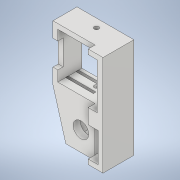
# Autodesk Inventor part: 30_Mount_Nema_Motor_attachement_for_XYstage_v3
Saved by Autodesk Inventor 2022.3 (Build 263350000, 350)
## iProperties
Created: 2021-05-10
Part Number: 30_Mount_Nema_Motor_attachement_for_XYstage_v3
Material: Generic
Document SubType Name: Modeling
Designer: diederichbenedict
Density: 1 g/cm^3
Appearance: Smooth - White
Author: diederichbenedict
Autodesk Inventor part; units mm, degrees
ref_plane "YZ Plane" through (0, 0, 0) normal (1, 0, 0) x (0, 1, 0)
sketch "Sketch1" plane through (0, 0, 0) normal (0, 0, 1) x (1, 0, 0)
  arc A0 (-7.9, -11.4) -> (-11.4, -7.9) centre (-11.4, -11.4) ccw projected
  line L0 (-7.9, -11.4) -> (-7.9, -13.5) projected
  line L1 (7.9, -13.5) -> (-7.9, -13.5) projected
  line L2 (7.9, -13.5) -> (7.9, -11.4) projected
  arc A1 (11.4, -7.9) -> (7.9, -11.4) centre (11.4, -11.4) ccw projected
  line L3 (11.4, -7.9) -> (13.5, -7.9) projected
  line L4 (13.5, 7.9) -> (13.5, -7.9) projected
  line L5 (13.5, 7.9) -> (11.4, 7.9) projected
  arc A2 (7.9, 11.4) -> (11.4, 7.9) centre (11.4, 11.4) ccw projected
  line L6 (7.9, 11.4) -> (7.9, 13.5) projected
  line L7 (-7.9, 13.5) -> (7.9, 13.5) projected
  line L8 (-7.9, 13.5) -> (-7.9, 11.4) projected
  arc A3 (-11.4, 7.9) -> (-7.9, 11.4) centre (-11.4, 11.4) ccw projected
  line L9 (-11.4, 7.9) -> (-13.5, 7.9) projected
  line L10 (-13.5, -7.9) -> (-13.5, 7.9) projected
  line L11 (-13.5, -7.9) -> (-11.4, -7.9) projected
  circle A4 centre (0, 0) radius 2.5 projected
  circle A5 centre (11.5, -26.7) radius 1.75 projected
  circle A6 centre (11.5, -38.3) radius 1.75 projected
  line L12 (14.7, -41.5) -> (14.7, -23.5) projected
  line L13 (14.7, -23.5) -> (8.7, -23.5) projected
  line L14 (8.7, -23.5) -> (8.7, -41.5) projected
  line L15 (8.7, -41.5) -> (14.7, -41.5) projected
  line L16 (-14, -11.5) -> (-14, -8.9) projected
  arc A7 (-14, -11.5) -> (-11.5, -14) centre (-11.5, -11.5) ccw projected
  line L17 (-8.9, -14) -> (-11.5, -14) projected
  line L18 (-8.9, -14) -> (-8.9, -11.4) projected
  arc A8 (-8.9, -11.4) -> (-11.4, -8.9) centre (-11.4, -11.4) ccw projected
  line L19 (-11.4, -8.9) -> (-14, -8.9) projected
  circle A9 centre (-11.5, -11.5) radius 1.1 projected
  arc A10 (-11.4, 8.9) -> (-8.9, 11.4) centre (-11.4, 11.4) ccw projected
  line L20 (-8.9, 11.4) -> (-8.9, 14) projected
  line L21 (-11.5, 14) -> (-8.9, 14) projected
  arc A11 (-11.5, 14) -> (-14, 11.5) centre (-11.5, 11.5) ccw projected
  line L22 (-14, 8.9) -> (-14, 11.5) projected
  line L23 (-14, 8.9) -> (-11.4, 8.9) projected
  circle A12 centre (-11.5, 11.5) radius 1.1 projected
  arc A13 (14, 11.5) -> (11.5, 14) centre (11.5, 11.5) ccw projected
  line L24 (14, 11.5) -> (14, 8.9) projected
  arc A14 (14, 11.5) -> (11.5, 14) centre (11.5, 11.5) ccw projected
  line L25 (8.9, 14) -> (11.5, 14) projected
  line L26 (8.9, 14) -> (8.9, 11.4) projected
  arc A15 (8.9, 11.4) -> (11.4, 8.9) centre (11.4, 11.4) ccw projected
  line L27 (11.4, 8.9) -> (14, 8.9) projected
  circle A16 centre (11.5, 11.5) radius 1.1 projected
  arc A17 (11.4, -8.9) -> (8.9, -11.4) centre (11.4, -11.4) ccw projected
  line L28 (8.9, -11.4) -> (8.9, -14) projected
  line L29 (11.5, -14) -> (8.9, -14) projected
  arc A18 (11.5, -14) -> (14, -11.5) centre (11.5, -11.5) ccw projected
  line L30 (14, -8.9) -> (14, -11.5) projected
  line L31 (14, -8.9) -> (11.4, -8.9) projected
  circle A19 centre (11.5, -11.5) radius 1.1 projected
  line L32 (8.6, -41.6) -> (8.6, -23.4)
  line L33 (8.6, -23.4) -> (14.8, -23.4)
  line L34 (14.8, -23.4) -> (14.8, -41.6)
  line L35 (14.8, -41.6) -> (8.6, -41.6)
  line L36 (-14, -14) -> (14, -14)
  line L37 (14, -14) -> (14, 13.7431)
  line L38 (14, 13.7431) -> (-14, 13.7431)
  line L39 (-14, 13.7431) -> (-14, -14)
  line L40 (-14.2, -14.2) -> (14.2, -14.2)
  line L41 (14.2, -14.2) -> (14.2, 13.9431)
  line L42 (14.2, 13.9431) -> (-14.2, 13.9431)
  line L43 (-14.2, 13.9431) -> (-14.2, -14.2)
  line L44 (-17.2, 17) -> (17.8, 17)
  line L45 (17.8, 17) -> (17.8, -44.6)
  line L46 (17.8, -44.6) -> (-9.3, -44.6)
  line L47 (-17.2, -17.2) -> (-17.2, 17)
  line L48 (-17.2, -17.2) -> (-9.3, -44.6)
  circle A20 centre (0, -32.5) radius 4.8 construction
  line L49 (8.7, -23.5) -> (-6.3, -23.5) construction
  line L50 (-6.3, -41.5) -> (-6.3, -23.5) construction
  line L51 (-6.3, -41.5) -> (8.7, -41.5) construction
  line L52 (8.7, -23.5) -> (8.7, -41.5) construction
  circle A21 centre (0, -32.5) radius 4.8 projected
  point P0 (0, 0)
  point P1 (-13.2125, 12.3229)
  dimension "d0" = 0.1
  dimension "d1" = 0.2
  dimension "d2" = 3
  dimension "d3" = 3
  dimension "d4" = 3
  dimension "d5" = 3
  dimension "d6" = 3
  dimension "d7" = 3
  constraints: 34 end point, 6 parallel, 3 perpendicular, 2 horizontal, 2 point on line, 7 other
  measures "d0" distance between parallel lines of L14 L32
  measures "d1" distance between parallel lines of L39 L43
  measures "d2" distance between parallel lines of L45 L34
  measures "d3" distance between parallel lines of L46 L35
  measures "d4" distance between parallel lines of L44 L25
  measures "d5" distance between parallel lines of L43 L47
  measures "d6" distance from line of L46.end L50
  measures "d7" distance from line of L47.start L40
ref_plane "Work Plane1" through (-6.3, -41.5, -8.6) normal (0, 0, 1) x (1, 0, 0)
extrude "Extrusion1" add sketch "Sketch1" against normal up to surface (8.6 mm away) contours L44 L45 L46 L48 L47
sketch "Sketch2" plane through (17.8, 17, -8.6) normal (0, 0, -1) x (-1, 0, 0)
  line L0 (8.9, -3.0569) -> (26.7, -3.0569) projected
  line L1 (26.7, -3.0569) -> (26.7, -3) projected
  line L2 (26.7, -3) -> (29.3, -3) projected
  arc A0 (29.8305, -3.0569) -> (29.3, -3) centre (29.3, -5.5) ccw projected
  line L3 (29.8305, -3.0569) -> (32, -3.0569) projected
  line L4 (32, -3.0569) -> (32, -31.2) projected
  line L5 (32, -31.2) -> (3.6, -31.2) projected
  line L6 (3.6, -31.2) -> (3.6, -3.0569) projected
  line L7 (3.6, -3.0569) -> (5.7695, -3.0569) projected
  arc A1 (6.3, -3) -> (5.7695, -3.0569) centre (6.3, -5.5) ccw projected
  line L8 (6.3, -3) -> (8.9, -3) projected
  line L9 (8.9, -3) -> (8.9, -3.0569) projected
  line L10 (9.2, -58.6) -> (3, -58.6) projected
  line L11 (3, -58.6) -> (3, -40.4) projected
  line L12 (3, -40.4) -> (9.2, -40.4) projected
  line L13 (9.2, -40.4) -> (9.2, -58.6) projected
  circle A2 centre (17.8, -49.5) radius 4.8 projected
  line L14 (35, -34.2) -> (35, 0) projected
  line L15 (35, 0) -> (0, 0) projected
  line L16 (0, 0) -> (0, -61.6) projected
  line L17 (0, -61.6) -> (27.1, -61.6) projected
  line L18 (27.1, -61.6) -> (35, -34.2) projected
  circle A3 centre (17.8, -49.5) radius 4.8 construction
  line L19 (3.1, -52.5) -> (9.1, -52.5) construction
  line L20 (9.1, -52.5) -> (9.1, -58.5) construction
  line L21 (9.1, -58.5) -> (24.1, -58.5) construction
  line L22 (24.1, -58.5) -> (24.1, -40.5) construction
  line L23 (24.1, -40.5) -> (9.1, -40.5) construction
  line L24 (9.1, -40.5) -> (9.1, -46.5) construction
  line L25 (9.1, -46.5) -> (3.1, -46.5) construction
  line L26 (3.1, -46.5) -> (3.1, -52.5) construction
  line L27 (3, -58.6) -> (24.7619, -58.6)
  line L28 (24.7619, -58.6) -> (24.7619, -40.4)
  line L29 (24.7619, -40.4) -> (3, -40.4)
  line L30 (3, -40.4) -> (3, -58.6)
  point P0 (17.8, -17)
  dimension "d10" = 18.2
  constraints: 8 end point, 2 parallel, 1 horizontal, 1 perpendicular, 1 point on line
  measures "d10" distance between parallel lines of L29 L27
ref_plane "Work Plane2" through (-6.3, -41.5, -19) normal (0, 0, -1) x (0, 1, 0)
extrude "Extrusion2" add sketch "Sketch2" along normal up to surface (10.4 mm away) contours L18 L17 L16 L15 L14
sketch "Sketch3" plane through (-17.2, -17.2, 0) normal (-1, 0, 0) x (0, 0, 1)
  line L0 (-31.5, 3.2) -> (-23.9, 3.2) projected
  line L1 (0, 3) -> (-19, 3) projected
  line L2 (-8.1, 3.2) -> (-2.4, 3.2) projected
  circle A0 centre (-9.8509, 1.8611) radius 1.4
  circle A1 centre (-16.162, 1.8611) radius 1.4
  point P0 (0, 17.2)
  dimension "d13" = 2.8
  dimension "d14" = 2.8
  constraints: 2 centre point
  measures "d13" diameter of A0
  measures "d14" diameter of A1
extrude "Extrusion3" cut sketch "Sketch3" against normal blind 20
sketch "Sketch4" plane through (-9.3, -44.6, 0) normal (0, -1, 0) x (1, 0, 0)
  circle A0 centre (9.3, -13.8) radius 1.4 projected
  line L0 (18, -19) -> (18, -13.0213) projected
  line L1 (18, -13.0213) -> (24, -13.0213) projected
  line L2 (24, 3) -> (24, -13.0213) projected
  line L3 (18, 3) -> (24, 3) projected
  line L4 (18, 3) -> (18, -8.6) projected
  line L5 (3, -8.6) -> (18, -8.6) projected
  line L6 (3, -19) -> (3, -8.6) projected
  line L7 (18, -19) -> (3, -19) projected
  line L8 (18, 3) -> (-9.7986, 3)
  line L9 (-9.7986, 3) -> (-9.7986, -4.2162)
  line L10 (-9.7986, -4.2162) -> (18, -4.2162)
  line L11 (18, -4.2162) -> (18, 3)
  point P0 (9.3, 0)
  constraints: 8 end point, 2 parallel, 1 horizontal, 1 perpendicular
extrude "Extrusion4" cut sketch "Sketch4" against normal up to surface (61.6 mm away) contours A0 | L4 L10 L9 L8
sketch "Sketch5" plane through (-17.2, -17.2, -19) normal (-1, 0, 0) x (0, 0, 1)
  line L0 (14.7838, 0) -> (14.7838, 34.2) projected
  line L1 (14.7838, 34.2) -> (0, 34.2) projected
  line L2 (0, 34.2) -> (0, 0) projected
  line L3 (14.7838, 0) -> (0, 0) projected
  circle A0 centre (9.1491, 1.8611) radius 1.4 projected
  circle A1 centre (2.838, 1.8611) radius 1.4 projected
  line L4 (18.5, 14.7) -> (-32.3, 14.7)
  line L5 (-4.9, 5.7) -> (-4.9, 28.7) projected
  line L6 (-12.5, 28.7) -> (-4.9, 28.7) projected
  line L7 (-12.5, 28.7) -> (-12.5, 5.7) projected
  line L8 (-12.5, 5.7) -> (-4.9, 5.7) projected
  line L9 (18.5, 19.7) -> (-32.3, 19.7)
  line L10 (-2.2146, 10.8391) -> (2.2146, 10.8391)
  line L11 (2.2146, 10.8391) -> (2.2146, 23.5609)
  line L12 (2.2146, 23.5609) -> (-2.2146, 23.5609)
  line L13 (-2.2146, 23.5609) -> (-2.2146, 10.8391)
  line L14 (0, -27.4) -> (0, 34.2) projected
  line L15 (-2.2146, 10.8391) -> (2.2146, 23.5609) construction
  line L16 (2.2146, 10.8391) -> (-2.2146, 23.5609) construction
  line L17 (18.0484, 9.5152) -> (11.5192, 9.5152)
  line L18 (11.5192, 9.5152) -> (11.5192, 24.8848)
  line L19 (11.5192, 24.8848) -> (18.0484, 24.8848)
  line L20 (18.0484, 24.8848) -> (18.0484, 9.5152)
  line L21 (14.7838, 0) -> (14.7838, 34.2) projected
  line L22 (18.0484, 9.5152) -> (11.5192, 24.8848) construction
  line L23 (11.5192, 9.5152) -> (18.0484, 24.8848) construction
  point P0 (19, 17.2)
  point P1 (0, 17.2)
  point P2 (14.7838, 17.2)
  constraints: 28 end point, 4 horizontal, 4 midpoint, 4 parallel, 2 perpendicular, 2 point on line, 4 other
extrude "Extrusion5" cut sketch "Sketch5" against normal blind 20 contours L17 L18 L4 L0 | L0 L4 L20 L17 | L4 L18 L9 L0 | L0 L9 L20 L4 | L9 L18 L19 L0 | L0 L19 L20 L9
body "Solid1"
